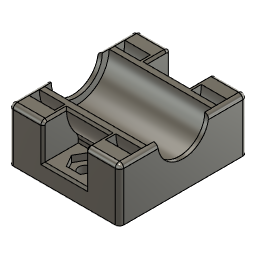
Bearing_holder_rev1 v10 (Autodesk Fusion 360 design; units mm, degrees)
Autodesk Fusion 360 part; units mm, degrees
sketch "Sketch1" plane through (0, 0, 0) normal (1, 0, 0) x (0, 0, -1)
  line L0 (0, 12.5) -> (0, 0)
  line L1 (0, 0) -> (-30, 0)
  line L2 (-30, 0) -> (-30, 12.5)
  arc A0 (-22.6, 12.5) -> (-7.4, 12.5) centre (-15, 12.5) ccw
  line L3 (-30, 12.5) -> (-22.6, 12.5)
  line L4 (-7.4, 12.5) -> (0, 12.5)
  dimension "d1" = 15.2
  dimension "d2" = 30
  dimension "d3" = 12.5
  constraint horizontal L3
  constraint vertical L0
  constraint horizontal L1
  constraint vertical L2
  constraint coincident L0.end L1.start
  constraint coincident A0.end L3
  constraint collinear L3 L4
  constraint coincident A0.centre L3
  constraint equal L3 L4
  measures "d1" diameter of A0
  measures "d2" horizontal distance of L0.end L1.end
  measures "d3" distance of L1 A0.centre
extrude "Extrude1" add sketch "Sketch1" along normal blind 26
sketch "Sketch2" plane through (26, 0, 0) normal (1, 0, 0) x (0, 0, -1)
  arc A0 (-22.6, 12.5) -> (-7.4, 12.5) centre (-15, 12.5) ccw
  line L0 (-22.6, 12.5) -> (-30, 12.5)
  line L1 (-30, 12.5) -> (-30, 0)
  line L2 (-30, 0) -> (0, 0)
  line L3 (0, 0) -> (0, 12.5)
  line L4 (0, 12.5) -> (-7.4, 12.5)
  line L5 (-22.6, 12.5) -> (-21, 12.5)
  line L6 (-9, 12.5) -> (-7.4, 12.5)
  arc A1 (-21, 12.5) -> (-9, 12.5) centre (-15, 12.5) ccw
  dimension "d6" = 12
  constraint concentric A0 A1
  constraint coincident A0.start L0.start
  constraint horizontal L5
  constraint coincident A0.end L4.end
  constraint parallel L5 L6
  measures "d6" diameter of A1
extrude "Extrude2" add sketch "Sketch2" against normal blind 0.95 contours A0 L5 L6 A1
sketch "Sketch3" plane through (0, 6.25, 15) normal (1, 0, 0) x (0, 0, -1)
  line L0 (7.6, 6.25) -> (15, 6.25)
  line L1 (6, 6.25) -> (7.6, 6.25)
  line L2 (-15, 6.25) -> (-7.6, 6.25)
  line L3 (-6, 6.25) -> (-7.6, 6.25)
  arc A0 (-6, 6.25) -> (6, 6.25) centre (0, 6.25) ccw
  arc A1 (-7.6, 6.25) -> (7.6, 6.25) centre (0, 6.25) ccw
  arc A2 (-7.6, 6.25) -> (7.6, 6.25) centre (0, 6.25) ccw
  point P0 (0, 6.25)
  dimension "d9" = 12
  constraint coincident P0 A0.centre
  constraint coincident L1.start A0.end
  constraint coincident L0.start L1.end
  constraint coincident L3.start A0.start
  constraint coincident L2.end L3.end
  measures "d9" diameter of A0
extrude "Extrude3" add sketch "Sketch3" along normal blind 0.95
ref_plane "WorkPlane1" through (22, 6.25, 15) normal (1, 0, 0) x (0, 0, -1)
fillet "Fillet1" radius 1 1 edges at (13, 12.5, 0)
fillet "Fillet2" radius 1 1 edges at (13, 12.5, 30)
sketch "Sketch6" plane through (0, 12.5, 0) normal (0, 1, 0) x (-1, 0, 0)
  line L0 (-26, 1) -> (0, 1)
  line L1 (0, 1) -> (0, 9)
  line L2 (0, 9) -> (-0.95, 9)
  line L3 (-0.95, 9) -> (-0.95, 7.4)
  line L4 (-0.95, 7.4) -> (-25.05, 7.4)
  line L5 (-25.05, 7.4) -> (-25.05, 9)
  line L6 (-25.05, 9) -> (-26, 9)
  line L7 (-26, 9) -> (-26, 1)
  circle A0 centre (-13, 5) radius 1.6
  circle A1 centre (-13, 25) radius 1.6
  line L8 (-13, 5) -> (-13, 25) construction
  line L9 (13, 15) -> (-39, 15) construction
  dimension "d15" = 3.2
  dimension "d16" = 3.2
  dimension "d17" = 20
  constraint coincident A0.centre L8.start
  constraint coincident A1.centre L8.end
  constraint symmetric A0 A1 L9
  measures "d15" diameter of A0
  measures "d16" diameter of A1
  measures "d17" vertical distance of A0.centre A1.centre
extrude "Extrude4" cut sketch "Sketch6" along normal blind -9 and the other way blind 30 contours A0 | A1
sketch "Sketch7" plane through (22, 6.25, 15) normal (1, 0, 0) x (0, 0, -1)
  arc A0 (-7.6, 6.25) -> (7.6, 6.25) centre (0, 6.25) ccw
  arc A1 (-7.6, 6.25) -> (7.6, 6.25) centre (0, 6.25) ccw
  line L0 (-15, 6.25) -> (-15, -6.25)
  line L1 (-15, -6.25) -> (15, -6.25)
  line L2 (15, -6.25) -> (15, 6.25)
  arc A2 (-10.05, 6.25) -> (10.05, 6.25) centre (0, 6.25) ccw
  line L3 (0, -1.35) -> (0, -3.8) construction
  line L4 (0, -3.8) -> (0, -6.25) construction
  arc A3 (-8.85, 6.2511) -> (8.85, 6.2511) centre (0, 6.2592) ccw
  arc A4 (-8.85, 6.2511) -> (-11.25, 6.2489) centre (-10.05, 6.25) ccw
  arc A5 (-11.25, 6.2489) -> (11.25, 6.2489) centre (0, 6.2592) ccw
  arc A6 (11.25, 6.2489) -> (8.85, 6.2511) centre (10.05, 6.25) ccw
  arc A7 (-10.05, 6.25) -> (10.05, 6.25) centre (0, 6.2592) ccw construction
  dimension "d22" = 1.2
  constraint coincident A0.centre A1.centre
  constraint horizontal A0.end A2.end
  constraint horizontal A0.start A2.start
  constraint midpoint A1 L3.start
  constraint midpoint A2 L3.end
  constraint midpoint L1 L4.end
  constraint equal L3 L4
  constraint tangent A3 A4
  constraint tangent A4 A5
  constraint tangent A5 A6
  constraint tangent A3 A6
  constraint coincident A2.end A6.centre
  constraint coincident A2.start A4.centre
  measures "d22" radius of A6
extrude "Extrude5" cut sketch "Sketch7" along normal mid plane 6
ref_plane "WorkPlane2" through (13, 12.5, 15) normal (1, 0, 0) x (0, 0, 1)
mirror "Mirror1" about plane through (13, 12.5, 15) normal (1, 0, 0) of "Extrude5"
ref_plane "WorkPlane3" through (13, 6.25, 15) normal (1, 0, 0) x (0, 0, -1)
sketch "Sketch9" plane through (13, 6.25, 15) normal (1, 0, 0) x (0, 0, -1)
  arc A0 (-6, 6.25) -> (6, 6.25) centre (0, 6.25) ccw
  arc A1 (-6, 6.25) -> (6, 6.25) centre (0, 6.25) ccw
  line L0 (-15, -2) -> (-15, -2.2)
  line L1 (-15, -2.2) -> (-6.7, -2.2)
  line L2 (0, -3.25) -> (0, -2)
  line L3 (-15, 5.25) -> (-15, -6.25)
  line L4 (15, -2) -> (15, -2.2)
  line L5 (15, -2.2) -> (6.7, -2.2)
  line L6 (0, -3.25) -> (0, -2)
  line L7 (-9.5, 6.25) -> (-15, 6.25)
  line L8 (-15, 6.25) -> (-15, -2)
  line L9 (9.5, 6.25) -> (15, 6.25)
  line L10 (15, 6.25) -> (15, -2)
  line L11 (6.7, -0.485) -> (6.7, -2.2)
  line L12 (-6.7, -0.485) -> (-6.7, -2.2)
  arc A2 (-9.5, 6.25) -> (-6.7, -0.485) centre (0, 6.25) ccw
  arc A3 (6.7, -0.485) -> (9.5, 6.25) centre (0, 6.25) ccw
  dimension "d34" = 19
  dimension "d44" = 8.3
  dimension "d45" = 8.3
  dimension "d50" = 0.2
  dimension "d51" = 0.2
  constraint concentric A1 A2
  constraint vertical L0
  constraint horizontal L1
  constraint vertical L2
  constraint coincident L0.end L3
  constraint vertical L4
  constraint horizontal L5
  constraint vertical L6
  constraint horizontal L7
  constraint vertical L8
  constraint horizontal L9
  constraint vertical L10
  constraint coincident L11.start A2
  constraint coincident L2.start A2
  constraint perpendicular L5 L11
  constraint perpendicular L1 L12
  constraint concentric A2 A3
  measures "d34" diameter of A2
  measures "d44" distance of L0 L12
  measures "d45" distance of L4 L11
  measures "d50" vertical distance of L0.start L0.end
  measures "d51" vertical distance of L4.start L4.end
extrude "Extrude8" cut sketch "Sketch9" along normal mid plane 10
sketch "Sketch11" plane through (0, 4.05, 0) normal (0, 1, 0) x (-1, 0, 0)
  line L0 (-8, 8.3) -> (-18, 8.3)
  line L1 (-18, 8.3) -> (-18, 0)
  line L2 (-8, 0) -> (-8, 8.3)
  line L3 (-9.7091, 25) -> (-11.3546, 27.85)
  line L4 (-11.3546, 27.85) -> (-14.6454, 27.85)
  line L5 (-14.6454, 27.85) -> (-16.2909, 25)
  line L6 (-16.2909, 25) -> (-14.6454, 22.15)
  line L7 (-14.6454, 22.15) -> (-11.3546, 22.15)
  line L8 (-11.3546, 22.15) -> (-9.7091, 25)
  circle A0 centre (-13, 25) radius 1.6 construction
  point P0 (-13, 25)
  dimension "d38" = 2.85
  constraint coincident P0 A0.centre
  constraint horizontal L3.start P0
  measures "d38" distance of P0 L8
extrude "Extrude9" cut sketch "Sketch11" against normal blind 1.5
sketch "Sketch12" plane through (0, 4.05, 0) normal (0, 1, 0) x (-1, 0, 0)
  line L0 (-8, 8.3) -> (-18, 8.3)
  line L1 (-18, 8.3) -> (-18, 0)
  line L2 (-18, 0) -> (-8, 0)
  line L3 (-8, 0) -> (-8, 8.3)
  line L4 (-15.85, 3.3546) -> (-13, 1.7091)
  line L5 (-13, 1.7091) -> (-10.15, 3.3546)
  line L6 (-10.15, 3.3546) -> (-10.15, 6.6454)
  line L7 (-10.15, 6.6454) -> (-13, 8.2909)
  line L8 (-13, 8.2909) -> (-15.85, 6.6454)
  line L9 (-15.85, 6.6454) -> (-15.85, 3.3546)
  point P0 (-13, 5)
  dimension "d41" = 2.85
  measures "d41" distance of P0 L9
extrude "Extrude10" cut sketch "Sketch12" against normal blind 1.5 contours L4 L5 L6 L7 L8 L9
chamfer "Chamfer1" distance 0.5 angle 45 8 edges at (18, 7.775, 0) (18, 12.2071, 0.2929) (18, 12.5, 3.25) (13, 12.5, 5.5) (8, 12.5, 3.25) (8, 12.2071, 0.2929) (8, 7.775, 0) (13, 4.05, 0)
chamfer "Chamfer2" distance 0.5 angle 45 8 edges at (8, 7.775, 30) (8, 12.2071, 29.7071) (8, 12.5, 26.75) (13, 12.5, 24.5) (18, 12.5, 26.75) (18, 12.2071, 29.7071) (18, 7.775, 30) (13, 4.05, 30)
fillet "Fillet3" radius 2 1 edges at (13, 5.765, 21.7)
fillet "Fillet4" radius 2 1 edges at (13, 5.765, 8.3)
fillet "Fillet5" radius 1 3 edges at (26, 12.5, 25) (26, 12.2071, 29.7071) (26, 5.75, 30)
fillet "Fillet6" radius 1 9 edges at (26, 5.75, 0) (26, 12.2071, 0.2929) (26, 12.5, 5) (0, 12.5, 5) (0, 12.2071, 0.2929) (0, 5.75, 0) (0, 5.75, 30) (0, 12.2071, 29.7071) (0, 12.5, 25)
ref_plane "WorkPlane4" through (13, 5.75, 15) normal (0, 0, 1) x (0, -1, 0)
equation "d7 = -wall_width"
equation "d10 = wall_width"
equation "wall_width = 0.95 mm"
equation "nut_depth = 3 mm"
